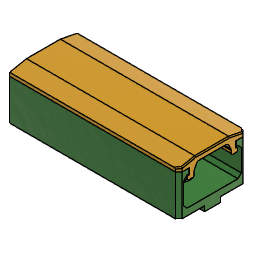
cnc3018_Kabelkanal v6 (Autodesk Fusion 360 design; units mm, degrees)
Autodesk Fusion 360 part; units mm, degrees
sketch "Skizze1" plane through (0, 0, 0) normal (1, 0, 0) x (0, 1, 0)
  line L0 (0, 0) -> (0, 25) construction
  line L1 (0, 0) -> (-10, 0)
  line L2 (-10, 0) -> (-10, 12)
  line L3 (-10, 12) -> (-7, 12)
  line L4 (-7, 12) -> (-7, 10.5)
  line L5 (-7, 10.5) -> (-8.5, 10.5)
  line L6 (-8.5, 10.5) -> (-8.5, 2)
  line L7 (-8.5, 2) -> (0, 2)
  line L8 (0, 0) -> (10, 0)
  line L9 (8.5, 2) -> (0, 2)
  line L10 (7, 10.5) -> (8.5, 10.5)
  line L11 (7, 12) -> (7, 10.5)
  line L12 (10, 0) -> (10, 12)
  line L13 (8.5, 10.5) -> (8.5, 2)
  line L14 (10, 12) -> (7, 12)
  line L15 (0, -1.5) -> (2.35, -1.5)
  line L16 (2.35, -1.5) -> (2.35, 0)
  line L17 (0, -1.5) -> (-2.35, -1.5)
  line L18 (-2.35, -1.5) -> (-2.35, 0)
  line L19 (-10, 12) -> (-10, 13)
  line L20 (-10, 13) -> (-5, 14)
  line L21 (-5, 14) -> (0, 14)
  line L22 (10, 12) -> (10, 13)
  line L23 (5, 14) -> (0, 14)
  line L24 (10, 13) -> (5, 14)
  line L25 (4.5, 12.5) -> (0, 12.5)
  line L26 (10, 12) -> (7, 12)
  line L27 (5.5, 10.5) -> (4.5, 12.5)
  line L28 (7, 12) -> (6.85, 12)
  line L29 (6.85, 12) -> (6.85, 10.5)
  line L30 (6.85, 10.5) -> (5.5, 10.5)
  line L31 (-7, 12) -> (-6.85, 12)
  line L32 (-6.85, 12) -> (-6.85, 10.5)
  line L33 (-6.85, 10.5) -> (-5.5, 10.5)
  line L34 (-5.5, 10.5) -> (-4.5, 12.5)
  line L35 (-4.5, 12.5) -> (0, 12.5)
  line L36 (6.85, 10.5) -> (6.85, 10.2)
  line L37 (6.85, 10.2) -> (7.4, 10.2)
  line L38 (7.4, 10.2) -> (7.4, 9)
  line L39 (7.4, 9) -> (5.5, 9)
  line L40 (5.5, 9) -> (5.5, 10.5)
  line L41 (-6.85, 10.5) -> (-6.85, 10.2)
  line L42 (-6.85, 10.2) -> (-7.4, 10.2)
  line L43 (-7.4, 10.2) -> (-7.4, 9)
  line L44 (-7.4, 9) -> (-5.5, 9)
  line L45 (-5.5, 9) -> (-5.5, 10.5)
  dimension "d1" = 20
  dimension "d3" = 14
  dimension "d4" = 1.5
  dimension "d5" = 2
  dimension "d6" = 1.5
  dimension "d7" = 12
  dimension "d11" = 1.5
  dimension "d12" = 4.7
  dimension "d13" = 2
  dimension "d14" = 1
  dimension "d17" = 13.7
  dimension "d18" = 9
  dimension "d19" = 1.5
  dimension "d21" = 11
  dimension "d27" = 0.3
  dimension "d28" = 0.4
  dimension "d29" = 1.5
  constraint coincident L0.start L1.start
  constraint vertical L0
  constraint perpendicular L0 L1
  constraint perpendicular L1 L2
  constraint perpendicular L2 L3
  constraint perpendicular L3 L4
  constraint perpendicular L3 L6
  constraint coincident L0 L7.end
  constraint perpendicular L0 L7
  constraint symmetric L1.start L0 L8.start
  constraint symmetric L0 L1.start L8.start
  constraint symmetric L0 L1.end L8.end
  constraint symmetric L0 L2.end L12.end
  constraint symmetric L0 L3.end L11.start
  constraint symmetric L0 L4.end L10.start
  constraint symmetric L0 L5.end L10.end
  constraint symmetric L0 L6.end L9.start
  constraint symmetric L0 L7.end L9.end
  constraint horizontal L15
  constraint coincident L8 L16.end
  constraint perpendicular L8 L16
  constraint symmetric L0 L15.start L17.start
  constraint symmetric L0 L15.end L17.end
  constraint symmetric L0 L16.end L18.end
  constraint perpendicular L3 L19
  constraint coincident L0 L21.end
  constraint perpendicular L0 L21
  constraint symmetric L0 L19.end L22.end
  constraint symmetric L0 L20.end L23.start
  constraint symmetric L0 L21.end L23.end
  constraint perpendicular L11 L28
  constraint perpendicular L28 L29
  constraint symmetric L0 L11.start L3.end
  constraint symmetric L0 L25.start L34.end
  constraint symmetric L0 L25.end L35.end
  constraint symmetric L0 L27.start L33.end
  constraint symmetric L0 L28.end L31.end
  constraint symmetric L0 L29.end L32.end
  constraint perpendicular L30 L36
  constraint perpendicular L36 L37
  constraint perpendicular L37 L38
  constraint perpendicular L38 L39
  constraint vertical L40
  constraint collinear L10 L30
  constraint symmetric L0 L36.end L41.end
  constraint symmetric L0 L37.end L42.end
  constraint symmetric L0 L38.end L43.end
  constraint symmetric L0 L39.end L44.end
  measures "d1" distance of L2 L12
  measures "d3" distance of L4 L11
  measures "d4" distance of L2 L6
  measures "d5" distance of L1 L7
  measures "d6" distance of L3 L5
  measures "d7" distance of L8 L14
  measures "d11" distance of L1 L17
  measures "d12" distance of L16 L18
  measures "d13" distance of L3 L21
  measures "d14" distance of L2.end L19.end
  measures "d17" distance of L29 L32
  measures "d18" distance of L25.start L34.end
  measures "d19" distance of L23 L25
  measures "d21" distance of L27.start L33.end
  measures "d27" distance of L10 L37
  measures "d28" distance of L11 L38
  measures "d29" distance of L30 L39
extrude "Extrusion1" add sketch "Skizze1" along normal blind 50 contours L1 L8 L15 L16 L17 L18 | L1 L2 L3 L4 L5 L6 L7 L8 L9 L10 L11 L12 L13 L14 L26 makes body 1
chamfer "Fase1" distance 1 angle 45 4 edges at (25, 8.5, 2) (25, -8.5, 2) (25, -8.5, 10.5) (25, 8.5, 10.5) on bodies 1
copy_body "Körper->Berechn1" bodies 1 removing the originals makes body 2 in component "Kabelkanal"
extrude "Extrusion1'" add sketch "Skizze1" along normal blind 50 separate body contours L3 L14 L19 L20 L21 L22 L23 L24 L25 L26 L27 L28 L29 L30 L31 L32 L33 L34 L35 | L33 L41 L42 L43 L44 L45 | L30 L36 L37 L38 L39 L40 makes body 3 in component "Kabelkanaldeckel"
sketch "Skizze1 (2)" plane through (0, 0, 2) normal (0, 0, 1) x (-1, 0, 0) in component "Kabelkanal"
  line L0 (0, 7.5) -> (-50, 7.5)
  line L1 (-50, 7.5) -> (-50, -7.5)
  line L2 (-50, -7.5) -> (0, -7.5)
  line L3 (0, -7.5) -> (0, 7.5)
  line L4 (0, 0) -> (-10, 0) construction
  circle A0 centre (-10, 0) radius 1.75
  circle A1 centre (-10, 0) radius 3.25
  line L5 (0, -10) -> (-50, -10)
  line L6 (0, 10) -> (-50, 10)
  line L7 (-25, -10) -> (-25, 10) construction
  circle A2 centre (-40, 0) radius 3.25
  circle A3 centre (-40, 0) radius 1.75
  dimension "d22" = 3.5
  dimension "d23" = 6.5
  dimension "d36" = 10
  constraint coincident L4.start origin
  constraint perpendicular L3 L4
  constraint coincident L4.end A0.centre
  constraint concentric A0 A1
  constraint midpoint L5 L7.start
  constraint midpoint L6 L7.end
  constraint symmetric A0 L7 A3
  constraint symmetric A1 L7 A2
  measures "d22" diameter of A0
  measures "d23" diameter of A1
  measures "d36" distance of L4.start L4.end
extrude "Extrusion1''" cut sketch "Skizze1 (2)" against normal through all contours A0 | A3 bodies 2 in component "Kabelkanal"
extrude "Extrusion2" cut sketch "Skizze1 (2)" against normal blind 1 contours A1 | A2 bodies 2 in component "Kabelkanal"
chamfer "Fase1'" distance 0.2 angle 45 2 edges at (25, 7.4, 10.2) (25, -7.4, 10.2) on bodies 3 in component "Kabelkanaldeckel"
fillet "Abrundung1" radius 0.5 4 edges at (25, 5.5, 9) (25, 7.4, 9) (25, -5.5, 9) (25, -7.4, 9) on bodies 3 in component "Kabelkanaldeckel"
fillet "Abrundung2" radius 1 4 edges at (25, -5.5, 10.5) (25, 5.5, 10.5) (25, 4.5, 12.5) (25, -4.5, 12.5) on bodies 3 in component "Kabelkanaldeckel"
chamfer "Fase1''" distance 0.2 angle 45 2 edges at (25, 7, 12) (25, -7, 12) on bodies 2 in component "Kabelkanal"
chamfer "Fase2" distance 1 angle 45 2 edges at (50, -10, 6) (50, 10, 6) on bodies 2 in component "Kabelkanal"
chamfer "Fase2'" distance 1 angle 45 2 edges at (50, -10, 12.5) (50, 10, 12.5) on bodies 3 in component "Kabelkanaldeckel"
chamfer "Fase3" distance 0.3 angle 45 5 edges at (49.5, -9.5, 13.1) (50, -7, 13.6) (50, 0, 14) (50, 7, 13.6) (49.5, 9.5, 13.1) on bodies 3 in component "Kabelkanaldeckel"
component "Kabelkanaldeckel" placed x (1, 0, 0) y (0, 1, 0) z (0, 0, 1) at (0, 0, 0)
component "Kabelkanal" placed x (1, 0, 0) y (0, 1, 0) z (0, 0, 1) at (0, 0, 0)
named bodies: "Kabelkanal"
